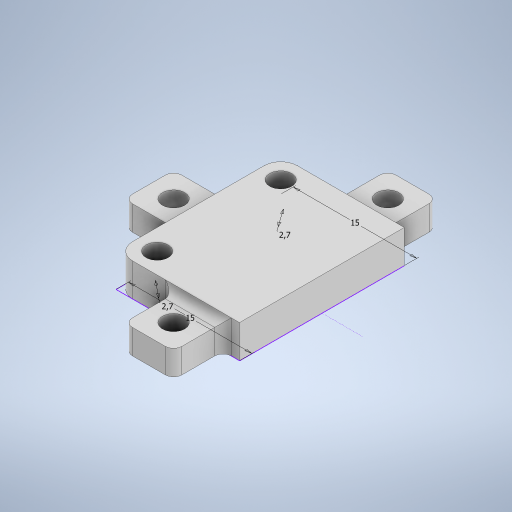
# Autodesk Inventor part: крепление_RGB
Saved by Autodesk Inventor 2023 (Build 270158000, 158)
## iProperties
Created: 2025-12-14
Part Number: крепление_RGB
Material: Типовые
Document SubType Name: Modeling
Designer: garin
Density: 1 g/cm^3
Appearance: По умолчанию
Author: garin
Autodesk Inventor part; units mm, degrees
ref_plane "YZ Plane" through (0, 0, 0) normal (1, 0, 0) x (0, 1, 0)
ref_plane "XZ Plane" through (0, 0, 0) normal (0, 1, 0) x (-1, 0, 0)
ref_plane "XY Plane" through (0, 0, 0) normal (0, 0, 1) x (1, 0, 0)
sketch "Эскиз1" plane through (0, 0, 0) normal (0, 1, 0) x (-1, 0, 0)
  line L0 (10, -10) -> (10, 10)
  line L1 (10, 0) -> (-10, 0) construction
  line L2 (0, -10) -> (0, 10) construction
  line L3 (10, -10) -> (9, -10) construction
  line L4 (10, -9) -> (10, -10) construction
  circle A0 centre (7.5, -7.5) radius 1.35
  circle A1 centre (7.5, 7.5) radius 1.35
  line L5 (10, -10) -> (-5, -10)
  line L6 (10, 10) -> (-5, 10)
  line L7 (-5, 10) -> (-5, -10)
  point P0 (0, 0)
  point P1 (0, 0)
  point P2 (0, 0)
  dimension "d16" = 2.7
  dimension "d17" = 2.7
  dimension "d25" = 15
  dimension "d26" = 15
  constraints: 16 end point, 3 horizontal, 3 midpoint, 2 centre point, 1 coincident, 1 perpendicular
  measures "d16" diameter of A0
  measures "d17" diameter of A1
  measures "d25" distance of L0.start L5.end
  measures "d26" distance of L0.end L6.end
extrude "Выдавливание1" add sketch "Эскиз1" along normal blind 4 contours L5 L7 L6 L0 | A0 | A1
sketch "Эскиз2" plane through (0, 0, 0) normal (0, -1, 0) x (1, 0, 0)
  line L0 (0, -10) -> (2.5, -10) construction
  line L1 (0, -10) -> (-3, -10)
  line L2 (-3, -10) -> (-3, -16)
  line L3 (-3, -16) -> (0, -16)
  line L4 (-3, -16) -> (3, -16)
  line L5 (3, -16) -> (3, -10)
  line L6 (3, -10) -> (-3, -10)
  line L7 (-3, -10) -> (-3, -16)
  line L8 (-10, -10) -> (-10, 10) construction
  line L9 (-10, 0) -> (5, 0) construction
  line L10 (5, 10) -> (5, -10) construction
  line L11 (0, 10) -> (2.5, 10) construction
  line L12 (0, 15) -> (0, 10) construction
  line L13 (0, 10) -> (-3, 10)
  line L14 (-3, 16) -> (0, 16)
  line L15 (-3, 16) -> (3, 16)
  line L16 (3, 16) -> (3, 10)
  line L17 (3, 10) -> (-3, 10)
  line L18 (5, -10) -> (5, 10) construction
  line L19 (-3, 16) -> (-3, 10)
  line L20 (-10, 10) -> (5, 10) construction
  line L21 (-2.5, 0) -> (-10, 10) construction
  line L22 (-10, 0) -> (-16, 0) construction
  line L23 (-16, 0) -> (-16, -3) construction
  line L24 (-16, -3) -> (-10, -3) construction
  line L25 (-10, -3) -> (-10, 0) construction
  line L26 (-10, -3) -> (-16, -3)
  line L27 (-16, -3) -> (-16, 3)
  line L28 (-16, 3) -> (-10, 3)
  line L29 (-10, 3) -> (-10, -3)
  circle A0 centre (-13, 0) radius 1.35
  circle A1 centre (0, 13) radius 1.35
  circle A2 centre (0, -13) radius 1.35
  point P0 (-2.5, -10)
  dimension "d30" = 6
  dimension "d31" = 6
  dimension "d33" = 6
  dimension "d34" = 3
  dimension "d35" = 6
  dimension "d39" = 2.7
  dimension "d40" = 2.7
  dimension "d41" = 2.7
  constraints: 54 end point, 10 symmetric about line, 7 parallel, 5 horizontal, 4 midpoint, 4 perpendicular, 3 centre point, 2 point on line, 1 vertical
  measures "d30" distance of L2.end L1.end
  measures "d31" distance of L6.end L5.end
  measures "d33" distance of L24.end L23.end
  measures "d34" distance of L23.end L22.end
  measures "d35" distance of L26.end L27.end
  measures "d39" diameter of A0
  measures "d40" diameter of A1
  measures "d41" diameter of A2
extrude "Выдавливание2" cut sketch "Эскиз1" along normal blind 4 contours A0 | A1
fillet "Сопряжение3" radius 2 2 edges at (-10, 2, 10) (-10, 2, -10)
extrude "Выдавливание4" add sketch "Эскиз2" against normal blind 3
fillet "Сопряжение6" radius 1 15 edges at (3, 1.5, 16) (3, 1.5, 10) (-3, 1.5, 16) (-3, 1.5, 10) (0, 3, 10) (-10, 1.5, 3) (-16, 1.5, 3) (-16, 1.5, -3) (-10, 1.5, -3) (-10, 3, 0) (-3, 1.5, -10) (0, 3, -10) (-3, 1.5, -16) (3, 1.5, -16) (3, 1.5, -10)
